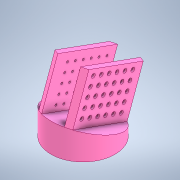
# Autodesk Inventor part: pvcBracketUpperPortionV02
Saved by Autodesk Inventor 2022.2 (Build 262287000, 287)
## iProperties
Created: 2021-10-20
Part Number: pvcBracketUpperPortionV02
Material: PC/ABS Plastic
Document SubType Name: Modeling
Designer: robst
Density: 0.357273 g/cm^3
Appearance: Pink
Author: robst
Autodesk Inventor part; units mm, degrees
ref_plane "YZ Plane" through (0, 0, 0) normal (1, 0, 0) x (0, 1, 0)
ref_plane "XZ Plane" through (0, 0, 0) normal (0, 1, 0) x (-1, 0, 0)
ref_plane "XY Plane" through (0, 0, 0) normal (0, 0, 1) x (1, 0, 0)
sketch "Sketch85" plane through (0, 0, 0) normal (0, 1, 0) x (-1, 0, 0)
  circle A0 centre (0, 0) radius 57.15
  dimension "d360" = 114.3
  constraints: 1 centre point, 1 coincident
  measures "d360" diameter of A0
extrude "Extrusion34" add sketch "Sketch85" along normal blind 60
sketch "Sketch86" plane through (0, 0, 0) normal (1, 0, 0) x (0, 1, 0)
  line L0 (0, 57.15) -> (60, 57.15) projected
  line L1 (0, -57.15) -> (0, 57.15) projected
  line L2 (60, -57.15) -> (60, 57.15) projected
  line L3 (0, -57.15) -> (60, -57.15) projected
  line L4 (51.6018, 57.15) -> (10, -57.15)
  line L5 (51.6018, 57.15) -> (51.6018, -57.15) construction
  point P0 (0, 0)
  dimension "d363" = 10
  dimension "d364" = 20
  constraints: 4 end point, 3 point on line, 1 perpendicular
  measures "d363" distance of L4.end L1.start
  measures "d364" angle of L4 L5
extrude "Extrusion35" cut sketch "Sketch86" along normal through all both and the other way through all contours L0 L2 L3 L4
sketch "Sketch90" plane through (0, 30.8009, 0) normal (0, 0.9396926, -0.3420201) x (1, 0, 0)
  ellipse E0 centre (0, 0) end of major axis (0, -60.8178) minor radius 57.15 projected
  line L0 (30.32, -51.553) -> (30.32, 51.553)
  line L1 (20.32, 56.8436) -> (20.32, -56.8436)
  arc A0 (30.32, 51.553) -> (20.32, 56.8436) centre (-1.2377, 4.0007) ccw
  arc A1 (20.32, -56.8436) -> (30.32, -51.553) centre (-1.2601, -3.9583) ccw
  point P0 (0, 10.5345)
  dimension "d378" = 10
  dimension "d379" = 20.32
  constraints: 4 end point, 4 point on circle, 2 centre point, 2 vertical, 5 other
  measures "d378" distance between parallel lines of L0 L1
  measures "d379" distance from line of L1 point (0, 0)
extrude "Extrusion38" add sketch "Sketch90" along normal blind 84.1375 contours A1 E0 | L1 A0 L0 A1 | E0 A0
mirror "Mirror6" about plane through (0, 0, 0) normal (1, 0, 0) of "Extrusion38"
sketch "Sketch91" plane through (-30.32, 13.1687, -48.444) normal (-1, 0, 0) x (0, 0.3420201, 0.9396926)
  line L0 (0, 0) -> (0, 84.1375) projected
  line L1 (0, 0) -> (103.106, 0) projected
  line L2 (10, 10) -> (103.106, 10) construction
  line L3 (10, 10) -> (10, 54.2582) construction
  point P0 (41.0185, -28.9434)
  point P1 (25, 10)
  point P2 (40, 10)
  point P3 (55, 10)
  point P4 (70, 10)
  point P5 (10, 25)
  point P6 (25, 25)
  point P7 (40, 25)
  point P8 (55, 25)
  point P9 (70, 25)
  point P10 (10, 40)
  point P11 (25, 40)
  point P12 (40, 40)
  point P13 (55, 40)
  point P14 (70, 40)
  point P15 (10, 55)
  point P16 (25, 55)
  point P17 (40, 55)
  point P18 (55, 55)
  point P19 (70, 55)
  point P20 (85, 10)
  point P21 (85, 25)
  point P22 (85, 40)
  point P23 (85, 55)
  point P24 (10, 70)
  point P25 (25, 70)
  point P26 (40, 70)
  point P27 (55, 70)
  point P28 (70, 70)
  point P29 (85, 70)
  dimension "d382" = 10
  dimension "d383" = 10
  dimension "d386" = 15
  dimension "d389" = 15
  constraints: 4 end point, 2 horizontal, 2 vertical, 29 other
  measures "d382" distance between parallel lines of L2 L1
  measures "d383" distance from line of L2.start L0
  measures "d386" distance of L2.start point (25, 10)
  measures "d389" distance of L2.start point (10, 25)
hole "Hole10" at (-30.32, 25.9859, -42.4673) at (-30.32, 31.1162, -28.3719) at (-30.32, 36.2465, -14.2765) at (-30.32, 41.3768, -0.1811) at (-30.32, 46.5071, 13.9143) at (-30.32, 40.0812, -47.5976) at (-30.32, 45.2115, -33.5022) at (-30.32, 50.3419, -19.4068) at (-30.32, 55.4722, -5.3114) at (-30.32, 60.6025, 8.784) at (-30.32, 54.1766, -52.7279) at (-30.32, 59.3069, -38.6325) at (-30.32, 64.4372, -24.5371) at (-30.32, 69.5675, -10.4417) at (-30.32, 74.6978, 3.6537) at (-30.32, 68.272, -57.8582) at (-30.32, 73.4023, -43.7628) at (-30.32, 78.5326, -29.6674) at (-30.32, 83.6629, -15.572) at (-30.32, 88.7932, -1.4766) at (-30.32, 82.3674, -62.9885) at (-30.32, 87.4977, -48.8931) at (-30.32, 92.628, -34.7977) at (-30.32, 97.7583, -20.7023) at (-30.32, 102.8886, -6.6069) at (-30.32, 108.0189, 7.4885) at (-30.32, 93.9235, 12.6188) at (-30.32, 79.8281, 17.7491) at (-30.32, 65.7328, 22.8794) at (-30.32, 51.6374, 28.0097) direction (1, 0, 0) diameter 3.797 depth 10 countersink diameter 7.087 countersink angle 82 clearance for "Flat Head Machine Screw (82)" size "#6" standard "Ansi Unified Screw Threads"
sketch "Sketch92" plane through (30.32, 48.4331, 48.444) normal (1, 0, 0) x (0, -0.3420201, -0.9396926)
  line L0 (0, 0) -> (0, 84.1375) projected
  line L1 (0, 0) -> (103.106, 0) projected
  line L2 (12, 14) -> (103.106, 14) construction
  line L3 (103.106, 0) -> (103.106, 84.1375) construction
  line L4 (12, 14) -> (12, 85.4375) construction
  point P0 (62.0875, -28.9434)
  point P1 (27, 14)
  point P2 (42, 14)
  point P3 (57, 14)
  point P4 (72, 14)
  point P5 (87, 14)
  point P6 (12, 29)
  point P7 (27, 29)
  point P8 (42, 29)
  point P9 (57, 29)
  point P10 (72, 29)
  point P11 (87, 29)
  point P12 (12, 44)
  point P13 (27, 44)
  point P14 (42, 44)
  point P15 (57, 44)
  point P16 (72, 44)
  point P17 (87, 44)
  point P18 (12, 59)
  point P19 (27, 59)
  point P20 (42, 59)
  point P21 (57, 59)
  point P22 (72, 59)
  point P23 (87, 59)
  point P24 (12, 74)
  point P25 (27, 74)
  point P26 (42, 74)
  point P27 (57, 74)
  point P28 (72, 74)
  point P29 (87, 74)
  dimension "d399" = 14
  dimension "d400" = 12
  dimension "d403" = 15
  dimension "d406" = 15
  constraints: 4 end point, 2 horizontal, 2 vertical, 1 point on line, 29 other
  measures "d399" distance from line of L2.start L1
  measures "d400" distance from line of L0 L2.start
  measures "d403" distance of L2.start point (27, 14)
  measures "d406" distance of L2.start point (12, 29)
hole "Hole11" at (30.32, 57.4845, 32.3794) at (30.32, 52.3542, 18.284) at (30.32, 47.2239, 4.1886) at (30.32, 42.0936, -9.9068) at (30.32, 36.9633, -24.0022) at (30.32, 31.833, -38.0976) at (30.32, 71.5799, 27.2491) at (30.32, 66.4496, 13.1537) at (30.32, 61.3193, -0.9417) at (30.32, 56.189, -15.0371) at (30.32, 51.0587, -29.1325) at (30.32, 45.9284, -43.2279) at (30.32, 85.6753, 22.1188) at (30.32, 80.545, 8.0234) at (30.32, 75.4147, -6.072) at (30.32, 70.2844, -20.1674) at (30.32, 65.1541, -34.2628) at (30.32, 60.0238, -48.3582) at (30.32, 99.7707, 16.9885) at (30.32, 94.6404, 2.8931) at (30.32, 89.5101, -11.2023) at (30.32, 84.3798, -25.2977) at (30.32, 79.2495, -39.3931) at (30.32, 74.1192, -53.4885) at (30.32, 113.8661, 11.8582) at (30.32, 108.7358, -2.2372) at (30.32, 103.6055, -16.3326) at (30.32, 98.4752, -30.428) at (30.32, 93.3449, -44.5234) at (30.32, 88.2146, -58.6188) direction (-1, 0, 0) diameter 3.797 depth 10 countersink diameter 7.087 countersink angle 82 clearance for "Flat Head Machine Screw (82)" size "#6" standard "Ansi Unified Screw Threads"
sketch "Sketch93" plane through (0, 0, 0) normal (0, -1, 0) x (1, 0, 0)
  point P0 (0, 0)
  point P1 (47.625, 0)
  point P2 (41.2445, 23.8125)
  point P3 (23.8125, 41.2445)
  point P4 (0, 47.625)
  point P5 (-23.8125, 41.2445)
  point P6 (-41.2445, 23.8125)
  point P7 (-47.625, 0)
  point P8 (-41.2445, -23.8125)
  point P9 (-23.8125, -41.2445)
  point P10 (0, -47.625)
  point P11 (23.8125, -41.2445)
  point P12 (41.2445, -23.8125)
  dimension "d416" = 47.625
  dimension "d419" = 360
  constraints: 13 other
  measures "d416" distance of point (47.625, 0) point (0, 0)
hole "Hole12" at (47.625, 0, 0) at (41.2445, 0, 23.8125) at (23.8125, 0, 41.2445) at (0, 0, 47.625) at (-23.8125, 0, 41.2445) at (-41.2445, 0, 23.8125) at (-47.625, 0, 0) at (-41.2445, 0, -23.8125) at (-23.8125, 0, -41.2445) at (0, 0, -47.625) at (23.8125, 0, -41.2445) at (41.2445, 0, -23.8125) direction (0, 1, 0) diameter 6.3754 depth 8 counterbore diameter 6.985 counterbore depth 5.7683
equation "\"twoByFourWidth\" = 40.64"
equation "\"twoByFourDepth\" = 84.1375"
equation "\"azimuth\" = 55deg"
equation "\"elevationOfTwoByFour\" = 20deg"
equation "\"depthOfExtrusionForMatingToLowerHalf\" = 12.5"
equation "\"depthForWasherForMatingToCase\" = 14"
equation "\"pvcPipeInsideDiameter\" = 50.8"
equation "\"pvcPipeOutsideDiameter\" = 2.375"
equation "\"pvcPipeInsertDepth\" = 25"
equation "\"outsideDiameterOfBottom\" = 88.9"
equation "\"angleForGarage2x4\" = 20deg"
body "Solid4"
body "Solid5"
